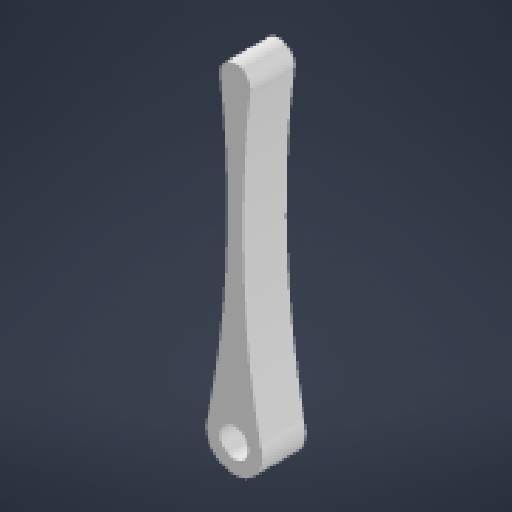
# Autodesk Inventor part: gate2
Saved by Autodesk Inventor 2026.2 (Build 302298000, 298)
## iProperties
Created: 2026-03-01
Part Number: gate2
Material: Generic
Document SubType Name: Modeling
Designer: danda
Density: 1 g/cm^3
Appearance: Default
Author: danda
Autodesk Inventor part; units mm, degrees
ref_plane "YZ Plane" through (0, 0, 0) normal (1, 0, 0) x (0, 1, 0)
ref_plane "XZ Plane" through (0, 0, 0) normal (0, 1, 0) x (-1, 0, 0)
ref_plane "XY Plane" through (0, 0, 0) normal (0, 0, 1) x (1, 0, 0)
sketch "Sketch1" plane through (0, 0, 0) normal (0, 0, 1) x (1, 0, 0)
  circle A0 centre (-1.3066, -22.8322) radius 2.3
  circle A1 centre (-1.3066, -22.8322) radius 4.5
  circle A2 centre (-1.1075, 27.1674) radius 2.5
  arc A3 (-5.8066, -22.8322) -> (-3.6075, 27.1674) centre (-152.4621, 8.6663) ccw
  arc A4 (1.3925, 27.1674) -> (3.1934, -22.8322) centre (150.0964, 7.4911) ccw
  point P0 (0, 0)
  point P1 (2.8463, -21.0992)
  point P2 (1.3093, 26.5276)
  point P3 (-3.5339, 26.5652)
  point P4 (-5.432, -21.0348)
  dimension "d0" = 4.6
  dimension "d1" = 9
  dimension "d2" = 5
  dimension "d3" = 50
  dimension "d17" = 150
  dimension "d18" = 150
  constraints: 8 point on circle, 5 centre point, 1 coincident
  measures "d0" diameter of A0
  measures "d1" diameter of A1
  measures "d2" diameter of A2
  measures "d3" distance of A0.centre A2.centre
  measures "d17" radius of A3
  measures "d18" radius of A4
extrude "Extrusion1" add sketch "Sketch1" along normal blind 5 and the other way blind 2
body "Solid1"
